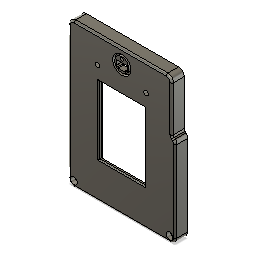
Caveatron Main Enclosure Lid v16 (Autodesk Fusion 360 design; units mm, degrees)
Autodesk Fusion 360 part; units mm, degrees
sketch "Sketch1" plane through (0, 0, 0) normal (0, 0, 1) x (1, 0, 0)
  arc A0 (6.35, 149.098) -> (3.302, 146.05) centre (6.35, 146.05) ccw
  line L0 (116.586, 156.21) -> (116.586, 152.4)
  line L1 (116.586, 152.4) -> (116.586, 105.4025)
  arc A1 (113.284, 105.4025) -> (115.1439, 100.9124) centre (119.634, 105.4025) ccw
  arc A2 (116.586, 105.4025) -> (117.4787, 103.2473) centre (119.634, 105.4025) ccw
  arc A3 (114.046, 0) -> (120.396, 6.35) centre (114.046, 6.35) ccw
  arc A4 (113.284, 146.017) -> (110.2512, 149.0649) centre (110.236, 146.017) ccw
  line L2 (97.5868, 6.35) -> (97.5868, 10.414)
  line L3 (6.35, 0) -> (23.495, 0)
  arc A5 (3.302, 16.51) -> (6.35, 13.462) centre (6.35, 16.51) ccw
  arc A6 (104.14, 156.21) -> (100.076, 160.274) centre (100.076, 156.21) ccw
  line L4 (120.396, 10.16) -> (120.396, 6.35)
  line L5 (117.4787, 103.2473) -> (118.5361, 102.1899)
  line L6 (110.236, 162.56) -> (103.886, 162.56)
  line L7 (0, 10.16) -> (0, 6.35)
  line L8 (22.8092, 6.35) -> (22.8092, 10.414)
  circle A7 centre (114.046, 6.35) radius 2.032
  arc A8 (114.3, 146.017) -> (110.2563, 150.0809) centre (110.236, 146.017) ccw
  arc A9 (114.046, 12.446) -> (118.11, 16.51) centre (114.046, 16.51) ccw
  line L9 (113.284, 146.017) -> (113.284, 105.4025)
  arc A10 (23.8252, 6.35) -> (26.8732, 3.302) centre (26.8732, 6.35) ccw
  line L10 (115.8623, 101.6308) -> (116.9197, 100.5734)
  arc A11 (116.586, 156.21) -> (110.236, 162.56) centre (110.236, 156.21) ccw
  circle A12 centre (110.236, 156.21) radius 3.81
  arc A13 (93.5228, 3.302) -> (96.5708, 6.35) centre (93.5228, 6.35) ccw
  arc A14 (22.8092, 6.35) -> (26.8732, 2.286) centre (26.8732, 6.35) ccw
  line L11 (116.586, 152.4) -> (116.586, 156.21)
  line L12 (0, 10.16) -> (0, 6.35)
  line L13 (104.14, 156.21) -> (104.14, 152.146)
  line L14 (120.396, 6.35) -> (120.396, 10.16)
  arc A15 (104.14, 152.146) -> (106.1619, 150.114) centre (106.172, 152.146) ccw
  circle A16 centre (6.35, 6.35) radius 2.032
  arc A17 (120.396, 97.6997) -> (118.5361, 102.1899) centre (114.046, 97.6997) ccw
  arc A18 (22.8092, 10.414) -> (20.7772, 12.446) centre (20.7772, 10.414) ccw
  arc A19 (0, 6.35) -> (6.35, 0) centre (6.35, 6.35) ccw
  line L15 (6.35, 0) -> (23.495, 0)
  line L16 (99.6188, 13.462) -> (114.046, 13.462)
  line L17 (20.7772, 13.462) -> (6.35, 13.462)
  arc A20 (114.3, 105.4025) -> (115.8623, 101.6308) centre (119.634, 105.4025) ccw
  arc A21 (103.124, 156.21) -> (100.076, 159.258) centre (100.076, 156.21) ccw
  line L18 (20.7772, 12.446) -> (6.35, 12.446)
  line L19 (110.2563, 150.0809) -> (106.1619, 150.114)
  line L20 (110.2512, 149.0649) -> (106.1568, 149.098)
  line L21 (96.901, 0) -> (114.046, 0)
  arc A22 (118.11, 97.6997) -> (116.9197, 100.5734) centre (114.046, 97.6997) ccw
  line L22 (103.124, 156.21) -> (103.124, 152.146)
  line L23 (23.8252, 6.35) -> (23.8252, 10.414)
  arc A23 (114.046, 13.462) -> (117.094, 16.51) centre (114.046, 16.51) ccw
  arc A24 (103.124, 152.146) -> (106.1568, 149.098) centre (106.172, 152.146) ccw
  arc A25 (99.6188, 12.446) -> (97.5868, 10.414) centre (99.6188, 10.414) ccw
  arc A26 (117.094, 97.6997) -> (116.2013, 99.855) centre (114.046, 97.6997) ccw
  arc A27 (99.6188, 13.462) -> (96.5708, 10.414) centre (99.6188, 10.414) ccw
  line L24 (115.1439, 100.9124) -> (116.2013, 99.855)
  line L25 (96.5708, 6.35) -> (96.5708, 10.414)
  line L26 (99.6188, 12.446) -> (114.046, 12.446)
  arc A28 (93.5228, 2.286) -> (97.5868, 6.35) centre (93.5228, 6.35) ccw
  line L27 (114.046, 0) -> (96.901, 0)
  arc A29 (2.286, 16.51) -> (6.35, 12.446) centre (6.35, 16.51) ccw
  line L28 (114.3, 146.017) -> (114.3, 105.4025)
  line L29 (26.8732, 3.302) -> (93.5228, 3.302)
  line L30 (23.495, 0) -> (96.901, 0)
  line L31 (26.8732, 2.286) -> (93.5228, 2.286)
  line L32 (110.236, 162.56) -> (103.886, 162.56)
  line L33 (118.11, 16.51) -> (118.11, 97.6997)
  line L34 (0, 152.4) -> (0, 10.16)
  line L35 (10.414, 150.114) -> (6.35, 150.114)
  line L36 (117.094, 16.51) -> (117.094, 97.6997)
  line L37 (10.16, 162.56) -> (6.35, 162.56)
  line L38 (3.302, 146.05) -> (3.302, 16.51)
  line L39 (100.076, 159.258) -> (16.51, 159.258)
  line L40 (2.286, 146.05) -> (2.286, 16.51)
  arc A30 (16.51, 160.274) -> (12.446, 156.21) centre (16.51, 156.21) ccw
  arc A31 (10.414, 149.098) -> (13.462, 152.146) centre (10.414, 152.146) ccw
  line L41 (10.414, 149.098) -> (6.35, 149.098)
  line L42 (0, 152.4) -> (0, 156.21)
  arc A32 (6.35, 150.114) -> (2.286, 146.05) centre (6.35, 146.05) ccw
  line L43 (13.462, 156.21) -> (13.462, 152.146)
  line L44 (0, 156.21) -> (0, 152.4)
  arc A33 (23.8252, 10.414) -> (20.7772, 13.462) centre (20.7772, 10.414) ccw
  line L45 (103.886, 162.56) -> (10.16, 162.56)
  line L46 (6.35, 162.56) -> (10.16, 162.56)
  arc A34 (16.51, 159.258) -> (13.462, 156.21) centre (16.51, 156.21) ccw
  line L47 (120.396, 10.16) -> (120.396, 97.6997)
  circle A35 centre (6.35, 156.21) radius 3.81
  line L48 (100.076, 160.274) -> (16.51, 160.274)
  arc A36 (10.414, 150.114) -> (12.446, 152.146) centre (10.414, 152.146) ccw
  arc A37 (6.35, 162.56) -> (0, 156.21) centre (6.35, 156.21) ccw
  line L49 (12.446, 156.21) -> (12.446, 152.146)
  line L50 (20.7772, 11.6332) -> (6.35, 11.6332)
  arc A38 (1.4732, 16.51) -> (6.35, 11.6332) centre (6.35, 16.51) ccw
  line L51 (1.4732, 146.05) -> (1.4732, 16.51)
  arc A39 (6.35, 150.9268) -> (1.4732, 146.05) centre (6.35, 146.05) ccw
  line L52 (10.414, 150.9268) -> (6.35, 150.9268)
  arc A40 (10.414, 150.9268) -> (11.6332, 152.146) centre (10.414, 152.146) ccw
  line L53 (11.6332, 156.21) -> (11.6332, 152.146)
  arc A41 (16.51, 161.0868) -> (11.6332, 156.21) centre (16.51, 156.21) ccw
  line L54 (100.076, 161.0868) -> (16.51, 161.0868)
  arc A42 (104.9528, 156.21) -> (100.076, 161.0868) centre (100.076, 156.21) ccw
  line L55 (104.9528, 156.21) -> (104.9528, 152.146)
  arc A43 (104.9528, 152.146) -> (106.165, 150.9268) centre (106.172, 152.146) ccw
  line L56 (110.2616, 150.8937) -> (106.165, 150.9268)
  arc A44 (115.1128, 146.017) -> (110.2616, 150.8937) centre (110.236, 146.017) ccw
  line L57 (115.1128, 146.017) -> (115.1128, 105.4025)
  arc A45 (115.1128, 105.4025) -> (116.437, 102.2056) centre (119.634, 105.4025) ccw
  line L58 (116.437, 102.2056) -> (117.4944, 101.1482)
  arc A46 (118.9228, 97.6997) -> (117.4944, 101.1482) centre (114.046, 97.6997) ccw
  line L59 (118.9228, 16.51) -> (118.9228, 97.6997)
  arc A47 (114.046, 11.6332) -> (118.9228, 16.51) centre (114.046, 16.51) ccw
  line L60 (99.6188, 11.6332) -> (114.046, 11.6332)
  arc A48 (99.6188, 11.6332) -> (98.3996, 10.414) centre (99.6188, 10.414) ccw
  line L61 (98.3996, 6.35) -> (98.3996, 10.414)
  arc A49 (93.5228, 1.4732) -> (98.3996, 6.35) centre (93.5228, 6.35) ccw
  line L62 (26.8732, 1.4732) -> (93.5228, 1.4732)
  arc A50 (21.9964, 6.35) -> (26.8732, 1.4732) centre (26.8732, 6.35) ccw
  line L63 (21.9964, 6.35) -> (21.9964, 10.414)
  arc A51 (21.9964, 10.414) -> (20.7772, 11.6332) centre (20.7772, 10.414) ccw
  line L64 (20.7772, 14.2494) -> (6.35, 14.2494)
  arc A52 (4.0894, 16.51) -> (6.35, 14.2494) centre (6.35, 16.51) ccw
  line L65 (4.0894, 146.05) -> (4.0894, 16.51)
  arc A53 (6.35, 148.3106) -> (4.0894, 146.05) centre (6.35, 146.05) ccw
  line L66 (10.414, 148.3106) -> (6.35, 148.3106)
  arc A54 (10.414, 148.3106) -> (14.2494, 152.146) centre (10.414, 152.146) ccw
  line L67 (14.2494, 156.21) -> (14.2494, 152.146)
  arc A55 (16.51, 158.4706) -> (14.2494, 156.21) centre (16.51, 156.21) ccw
  line L68 (100.076, 158.4706) -> (16.51, 158.4706)
  arc A56 (102.3366, 156.21) -> (100.076, 158.4706) centre (100.076, 156.21) ccw
  line L69 (102.3366, 156.21) -> (102.3366, 152.146)
  arc A57 (102.3366, 152.146) -> (106.1516, 148.3107) centre (106.172, 152.146) ccw
  line L70 (110.2461, 148.2776) -> (106.1516, 148.3107)
  arc A58 (112.4966, 146.017) -> (110.2461, 148.2776) centre (110.236, 146.017) ccw
  line L71 (112.4966, 146.017) -> (112.4966, 105.4025)
  arc A59 (112.4966, 105.4025) -> (114.5871, 100.3556) centre (119.634, 105.4025) ccw
  line L72 (114.5871, 100.3556) -> (115.6445, 99.2982)
  arc A60 (116.3066, 97.6997) -> (115.6445, 99.2982) centre (114.046, 97.6997) ccw
  line L73 (116.3066, 16.51) -> (116.3066, 97.6997)
  arc A61 (114.046, 14.2494) -> (116.3066, 16.51) centre (114.046, 16.51) ccw
  line L74 (99.6188, 14.2494) -> (114.046, 14.2494)
  arc A62 (99.6188, 14.2494) -> (95.7834, 10.414) centre (99.6188, 10.414) ccw
  line L75 (95.7834, 6.35) -> (95.7834, 10.414)
  arc A63 (93.5228, 4.0894) -> (95.7834, 6.35) centre (93.5228, 6.35) ccw
  line L76 (26.8732, 4.0894) -> (93.5228, 4.0894)
  arc A64 (24.6126, 6.35) -> (26.8732, 4.0894) centre (26.8732, 6.35) ccw
  line L77 (24.6126, 6.35) -> (24.6126, 10.414)
  arc A65 (24.6126, 10.414) -> (20.7772, 14.2494) centre (20.7772, 10.414) ccw
  line L78 (20.7772, 16.4338) -> (6.35, 16.4338)
  arc A66 (6.2738, 16.51) -> (6.35, 16.4338) centre (6.35, 16.51) ccw
  line L79 (6.2738, 146.05) -> (6.2738, 16.51)
  arc A67 (6.35, 146.1262) -> (6.2738, 146.05) centre (6.35, 146.05) ccw
  line L80 (10.414, 146.1262) -> (6.35, 146.1262)
  arc A68 (10.414, 146.1262) -> (16.4338, 152.146) centre (10.414, 152.146) ccw
  line L81 (16.4338, 156.21) -> (16.4338, 152.146)
  arc A69 (16.51, 156.2862) -> (16.4338, 156.21) centre (16.51, 156.21) ccw
  line L82 (100.076, 156.2862) -> (16.51, 156.2862)
  arc A70 (100.1522, 156.21) -> (100.076, 156.2862) centre (100.076, 156.21) ccw
  line L83 (100.1522, 156.21) -> (100.1522, 152.146)
  arc A71 (100.1522, 152.146) -> (106.1366, 146.1263) centre (106.172, 152.146) ccw
  line L84 (110.2351, 146.0932) -> (106.1366, 146.1263)
  arc A72 (110.3122, 146.017) -> (110.2351, 146.0932) centre (110.236, 146.017) ccw
  line L85 (110.3122, 146.017) -> (110.3122, 105.4025)
  arc A73 (110.3122, 105.4025) -> (113.0425, 98.811) centre (119.634, 105.4025) ccw
  line L86 (113.0425, 98.811) -> (114.0999, 97.7536)
  arc A74 (114.1222, 97.6997) -> (114.0999, 97.7536) centre (114.046, 97.6997) ccw
  line L87 (114.1222, 16.51) -> (114.1222, 97.6997)
  arc A75 (114.046, 16.4338) -> (114.1222, 16.51) centre (114.046, 16.51) ccw
  line L88 (99.6188, 16.4338) -> (114.046, 16.4338)
  arc A76 (99.6188, 16.4338) -> (93.599, 10.414) centre (99.6188, 10.414) ccw
  line L89 (93.599, 6.35) -> (93.599, 10.414)
  arc A77 (93.5228, 6.2738) -> (93.599, 6.35) centre (93.5228, 6.35) ccw
  line L90 (26.8732, 6.2738) -> (93.5228, 6.2738)
  arc A78 (26.797, 6.35) -> (26.8732, 6.2738) centre (26.8732, 6.35) ccw
  line L91 (26.797, 6.35) -> (26.797, 10.414)
  arc A79 (26.797, 10.414) -> (20.7772, 16.4338) centre (20.7772, 10.414) ccw
  circle A80 centre (60.198, 146.558) radius 7.9502
  circle A81 centre (60.198, 146.558) radius 10.287
  circle A82 centre (60.198, 151.892) radius 1.8796
  line L92 (53.848, 148.59) -> (66.548, 148.59)
  line L93 (66.548, 148.59) -> (66.548, 142.748)
  line L94 (66.548, 142.748) -> (53.848, 142.748)
  line L95 (53.848, 142.748) -> (53.848, 148.59)
  circle A83 centre (32.766, 132.588) radius 2.6162
  circle A84 centre (87.63, 132.588) radius 2.6162
  line L96 (6.2738, 126.238) -> (110.3122, 126.238)
  line L97 (34.29, 117.348) -> (86.106, 117.348)
  line L98 (86.106, 117.348) -> (86.106, 41.148)
  line L99 (86.106, 41.148) -> (34.29, 41.148)
  line L100 (34.29, 41.148) -> (34.29, 117.348)
  line L101 (88.646, 38.608) -> (31.75, 38.608)
  line L102 (31.75, 38.608) -> (31.75, 119.888)
  line L103 (31.75, 119.888) -> (88.646, 119.888)
  line L104 (88.646, 119.888) -> (88.646, 38.608)
  circle A85 centre (30.226, 122.428) radius 1.27
  circle A86 centre (90.17, 122.428) radius 1.27
  circle A87 centre (30.226, 27.94) radius 1.27
  circle A88 centre (90.17, 27.94) radius 1.27
  line L105 (31.75, 38.608) -> (88.646, 38.608)
  line L106 (88.646, 38.608) -> (88.646, 33.02)
  line L107 (88.646, 33.02) -> (31.75, 33.02)
  line L108 (31.75, 33.02) -> (31.75, 38.608)
  line L109 (26.416, 126.238) -> (26.416, 24.13)
  line L110 (93.98, 126.238) -> (93.98, 24.13)
  line L111 (34.29, 33.02) -> (34.29, 24.13)
  line L112 (34.29, 24.13) -> (26.416, 24.13)
  line L113 (86.106, 33.02) -> (86.106, 24.13)
  line L114 (86.106, 24.13) -> (93.98, 24.13)
  line L115 (34.29, 24.13) -> (86.106, 24.13)
  circle A89 centre (25.146, 84.328) radius 1.27
  circle A90 centre (95.25, 84.328) radius 1.27
  arc A91 (25.146, 88.138) -> (25.146, 80.518) centre (25.146, 84.328) ccw
  line L116 (25.146, 84.328) -> (25.146, 88.138) construction
  line L117 (25.146, 84.328) -> (25.146, 80.518) construction
  arc A92 (95.25, 80.518) -> (95.25, 88.138) centre (95.25, 84.328) ccw
  line L118 (95.25, 84.328) -> (95.25, 80.518) construction
  line L119 (95.25, 84.328) -> (95.25, 88.138) construction
  line L120 (95.25, 80.518) -> (93.98, 80.518)
  line L121 (95.25, 88.138) -> (93.98, 88.138)
  line L122 (25.146, 88.138) -> (26.416, 88.138)
  line L123 (25.146, 80.518) -> (26.416, 80.518)
  line L124 (34.29, 18.542) -> (86.106, 18.542)
  line L125 (86.106, 18.542) -> (86.106, 8.382)
  line L126 (86.106, 8.382) -> (34.29, 8.382)
  line L127 (34.29, 8.382) -> (34.29, 18.542)
  line L128 (26.416, 24.13) -> (26.416, 12.5216)
  line L129 (34.29, 24.13) -> (34.29, 18.542)
  line L130 (86.106, 24.13) -> (86.106, 18.542)
  line L131 (93.98, 24.13) -> (93.98, 12.5216)
  line L132 (34.29, 32.004) -> (86.106, 32.004)
  line L133 (81.28, 138.938) -> (93.98, 138.938)
  line L134 (93.98, 138.938) -> (93.98, 126.238)
  line L135 (93.98, 126.238) -> (81.28, 126.238)
  line L136 (81.28, 126.238) -> (81.28, 138.938)
  line L137 (81.28, 138.938) -> (93.98, 126.238) construction
  line L138 (93.98, 138.938) -> (81.28, 126.238) construction
  line L139 (26.416, 138.938) -> (39.116, 138.938)
  line L140 (39.116, 138.938) -> (39.116, 126.238)
  line L141 (39.116, 126.238) -> (26.416, 126.238)
  line L142 (26.416, 126.238) -> (26.416, 138.938)
  line L143 (26.416, 138.938) -> (39.116, 126.238) construction
  line L144 (39.116, 138.938) -> (26.416, 126.238) construction
  circle A93 centre (114.046, 6.35) radius 3.81
  circle A94 centre (6.35, 6.35) radius 3.81
  line L145 (64.262, 142.748) -> (56.134, 142.748)
  line L146 (56.134, 142.748) -> (56.134, 141.224)
  line L147 (56.134, 141.224) -> (64.262, 141.224)
  line L148 (64.262, 141.224) -> (64.262, 142.748)
  point P0 (87.63, 132.588)
  point P1 (32.766, 132.588)
  dimension "d2" = 10.16
  dimension "d3" = 23.495
  dimension "d5" = 6.35
  dimension "d6" = 3.048
  dimension "d7" = 6.35
  dimension "d8" = 6.35
  dimension "d9" = 6.35
  dimension "d10" = 6.35
  dimension "d11" = 3.048
  dimension "d12" = 3.048
  dimension "d13" = 3.048
  dimension "d14" = 3.048
  dimension "d15" = 3.048
  dimension "d16" = 3.048
  dimension "d17" = 3.048
  dimension "d18" = 3.048
  dimension "d19" = 3.048
  dimension "d20" = 3.048
  dimension "d21" = 3.048
  dimension "d22" = 3.048
  dimension "d30" = 7.62
  dimension "d31" = 7.62
  dimension "d32" = 4.064
  dimension "d33" = 4.064
  dimension "d40" = 0.8128
  dimension "d41" = -0.7874
  dimension "d42" = -2.9718
  dimension "d43" = 15.9004
  dimension "d44" = 60.198
  dimension "d45" = 16.002
  dimension "d46" = 2.3368
  dimension "d47" = 3.7592
  dimension "d48" = 5.334
  dimension "d49" = 12.7
  dimension "d50" = 5.842
  dimension "d51" = 6.35
  dimension "d52" = 3.302
  dimension "d53" = 5.2324
  dimension "d54" = 32.766
  dimension "d55" = 5.2324
  dimension "d56" = 54.864
  dimension "d57" = 29.972
  dimension "d58" = 29.972
  dimension "d59" = 36.322
  dimension "d60" = 51.816
  dimension "d61" = 76.2
  dimension "d62" = 34.29
  dimension "d63" = 41.148
  dimension "d64" = -2.54
  dimension "d65" = 2.54
  dimension "d66" = 4.064
  dimension "d67" = 5.08
  dimension "d68" = 2.54
  dimension "d69" = 4.064
  dimension "d70" = 5.08
  dimension "d71" = 2.54
  dimension "d72" = 4.064
  dimension "d73" = 13.208
  dimension "d74" = 2.54
  dimension "d75" = 13.208
  dimension "d76" = 4.064
  dimension "d77" = 5.588
  dimension "d78" = 102.108
  dimension "d79" = 7.874
  dimension "d80" = 102.108
  dimension "d81" = 7.874
  dimension "d82" = 2.54
  dimension "d83" = 33.02
  dimension "d84" = 9.144
  dimension "d85" = 2.54
  dimension "d86" = 33.02
  dimension "d87" = 9.144
  dimension "d88" = 3.81
  dimension "d89" = 180
  dimension "d90" = 3.81
  dimension "d91" = 180
  dimension "d92" = 10.16
  dimension "d93" = 5.08
  dimension "d108" = 4.064
  dimension "d121" = 12.7
  dimension "d122" = 12.7
  dimension "d123" = 12.7
  dimension "d124" = 12.7
  dimension "d132" = 7.62
  dimension "d133" = 7.62
  dimension "d170" = 8.128
  dimension "d171" = 1.524
  dimension "d172" = 2.286
  dimension "d175" = 26.797
  dimension "d176" = 26.797
  constraint horizontal L15
  constraint vertical L14
  constraint horizontal L6
  constraint vertical L44
  constraint vertical L0
  constraint horizontal L46
  constraint vertical L42
  constraint horizontal L32
  constraint vertical L11
  constraint horizontal L3
  constraint vertical L12
  constraint horizontal L27
  constraint vertical L4
  constraint tangent L5 A17
  constraint tangent A17 L47
  constraint tangent A2 L5
  constraint tangent L1 A2
  constraint tangent L6 A11
  constraint tangent L0 A11
  constraint tangent L46 A37
  constraint tangent L44 A37
  constraint tangent A3 L27
  constraint tangent A3 L4
  constraint tangent L3 A19
  constraint tangent L7 A19
  constraint parallel L34 L38
  constraint parallel L29 L30
  constraint parallel L36 L47
  constraint concentric A17 A26
  constraint parallel L5 L24
  constraint concentric A1 A2
  constraint parallel L1 L9
  constraint parallel L39 L45
  constraint tangent A26 L24
  constraint tangent A1 L9
  constraint tangent A1 L24
  constraint tangent A26 L36
  constraint tangent A0 L38
  constraint tangent A0 L41
  constraint tangent A31 L41
  constraint tangent A31 L43
  constraint tangent L43 A34
  constraint tangent L39 A34
  constraint tangent A21 L39
  constraint tangent A21 L22
  constraint tangent L22 A24
  constraint tangent A4 L9
  constraint tangent L16 A23
  constraint tangent A23 L36
  constraint tangent L16 A27
  constraint tangent A27 L25
  constraint tangent A13 L29
  constraint tangent A13 L25
  constraint tangent A10 L29
  constraint tangent A10 L23
  constraint tangent L17 A33
  constraint tangent L23 A33
  constraint tangent A5 L17
  constraint tangent A5 L38
  constraint parallel L17 L18
  constraint concentric A5 A29
  constraint parallel L38 L40
  constraint concentric A0 A32
  constraint parallel L35 L41
  constraint concentric A31 A36
  constraint parallel L43 L49
  constraint concentric A30 A34
  constraint parallel L39 L48
  constraint concentric A6 A21
  constraint parallel L13 L22
  constraint concentric A15 A24
  constraint concentric A4 A8
  constraint parallel L9 L28
  constraint concentric A1 A20
  constraint parallel L10 L24
  constraint concentric A22 A26
  constraint parallel L33 L36
  constraint concentric A9 A23
  constraint parallel L16 L26
  constraint concentric A25 A27
  constraint parallel L2 L25
  constraint concentric A13 A28
  constraint parallel L29 L31
  constraint concentric A10 A14
  constraint parallel L8 L23
  constraint concentric A18 A33
  constraint tangent L8 A18
  constraint tangent L8 A14
  constraint tangent A28 L31
  constraint tangent L2 A28
  constraint tangent A9 L26
  constraint tangent A9 L33
  constraint tangent L10 A22
  constraint tangent A25 L26
  constraint tangent L10 A20
  constraint tangent A29 L40
  constraint tangent A6 L13
  constraint tangent A30 L48
  constraint tangent L13 A15
  constraint tangent A36 L49
  constraint tangent A6 L48
  constraint tangent A22 L33
  constraint tangent L2 A25
  constraint tangent A14 L31
  constraint tangent L35 A36
  constraint tangent L35 A32
  constraint tangent L40 A32
  constraint tangent L18 A29
  constraint tangent A8 L28
  constraint tangent A30 L49
  constraint tangent A20 L28
  constraint tangent A18 L18
  constraint concentric A35 A37
  constraint concentric A11 A12
  constraint concentric A3 A7
  constraint concentric A16 A19
  constraint horizontal L92
  constraint vertical L93
  constraint horizontal L94
  constraint vertical L95
  constraint coincident L79 L96.start
  constraint coincident L85 L96.end
  constraint perpendicular L85 L96
  constraint horizontal L97
  constraint vertical L98
  constraint horizontal L99
  constraint vertical L100
  constraint horizontal L105
  constraint vertical L106
  constraint horizontal L107
  constraint vertical L108
  constraint coincident L96 L109.start
  constraint perpendicular L96 L109
  constraint coincident L96 L110.start
  constraint perpendicular L96 L110
  constraint coincident L107 L111.start
  constraint perpendicular L107 L111
  constraint perpendicular L109 L112
  constraint coincident L107 L113.start
  constraint perpendicular L107 L113
  constraint perpendicular L110 L114
  constraint coincident A89.centre A91.centre
  constraint coincident A90.centre A92.centre
  constraint coincident L110 L120.end
  constraint tangent A92 L120
  constraint perpendicular L110 L120
  constraint coincident L110 L121.end
  constraint tangent A92 L121
  constraint coincident L109 L122.end
  constraint tangent A91 L122
  constraint perpendicular L109 L122
  constraint coincident L109 L123.end
  constraint tangent A91 L123
  constraint horizontal L124
  constraint vertical L125
  constraint horizontal L126
  constraint vertical L127
  constraint coincident A79 L128.end
  constraint perpendicular L112 L128
  constraint perpendicular L124 L129
  constraint perpendicular L124 L130
  constraint coincident A76 L131.end
  constraint perpendicular L114 L131
  constraint coincident L111 L132.start
  constraint coincident L113 L132.end
  constraint perpendicular L113 L132
  constraint perpendicular L133 L134
  constraint parallel L133 L135
  constraint parallel L134 L136
  constraint horizontal L133
  constraint coincident L137 L3 P0
  constraint coincident L138 P0
  constraint coincident P0 A84.centre
  constraint perpendicular L139 L140
  constraint parallel L139 L141
  constraint parallel L140 L142
  constraint horizontal L139
  constraint coincident L143 P1
  constraint coincident L144 P1
  constraint coincident P1 A83.centre
  constraint concentric A7 A93
  constraint concentric A19 A94
  constraint horizontal L145
  constraint vertical L146
  constraint horizontal L147
  constraint vertical L148
  constraint coincident L94 L145.start
  measures "d2" distance of L7.start origin
  measures "d3" distance of L3.end origin
  measures "d5" radius of A17
  measures "d6" radius of A2
  measures "d7" radius of A11
  measures "d8" radius of A37
  measures "d9" radius of A3
  measures "d10" radius of A19
  measures "d11" radius of A0
  measures "d12" radius of A31
  measures "d13" radius of A34
  measures "d14" radius of A21
  measures "d15" radius of A24
  measures "d16" radius of A4
  measures "d17" radius of A23
  measures "d18" radius of A27
  measures "d19" radius of A13
  measures "d20" radius of A10
  measures "d21" radius of A33
  measures "d22" radius of A5
  measures "d30" diameter of A35
  measures "d31" diameter of A12
  measures "d32" diameter of A7
  measures "d33" diameter of A16
  measures "d43" diameter of A80
  measures "d44" distance of L34 A80.centre
  measures "d45" distance of L45 A80.centre
  measures "d47" diameter of A82
  measures "d48" distance of A80.centre A82.centre
  measures "d49" distance of L92.start L92.end
  measures "d50" distance of L92.start L94.end
  measures "d51" distance of A80.centre L93
  measures "d52" distance of A82.centre L92
  measures "d53" diameter of A83
  measures "d54" distance of L34 P1
  measures "d55" diameter of A84
  measures "d56" horizontal distance of P1 P0
  measures "d57" distance of L45 P1
  measures "d58" distance of L45 P0
  measures "d59" distance of L45 L96
  measures "d60" distance of L97.start L97.end
  measures "d61" distance of L97.start L99.end
  measures "d62" distance of L34 L100
  measures "d63" distance of L30 L99
  measures "d65" diameter of A85
  measures "d66" distance of L100 A85.centre
  measures "d67" distance of L97 A85.centre
  measures "d68" diameter of A86
  measures "d69" distance of L98 A86.centre
  measures "d70" distance of L97 A86.centre
  measures "d71" diameter of A87
  measures "d72" distance of L100 A87.centre
  measures "d73" distance of L99 A87.centre
  measures "d74" diameter of A88
  measures "d75" distance of L99 A88.centre
  measures "d76" distance of L98 A88.centre
  measures "d77" distance of L101.end L107.end
  measures "d78" distance of L109.start L109.end
  measures "d79" distance of L100 L109
  measures "d80" distance of L110.start L110.end
  measures "d81" distance of L98 L110
  measures "d82" diameter of A89
  measures "d83" distance of L97 A89.centre
  measures "d84" distance of L100 A89.centre
  measures "d85" diameter of A90
  measures "d86" distance of L97 A90.centre
  measures "d87" distance of L98 A90.centre
  measures "d88" radius of A91
  measures "d89" angle of L116 L117
  measures "d90" radius of A92
  measures "d91" angle of L118 L119
  measures "d92" distance of L124.start L126.end
  measures "d93" distance of L17 L124
  measures "d108" distance of A87.centre L132
  measures "d121" distance of L110.start L135.end
  measures "d122" distance of L133.end L110.start
  measures "d123" distance of L140.end L109.start
  measures "d124" distance of L139.end L140.end
  measures "d132" diameter of A93
  measures "d133" diameter of A94
  measures "d170" distance of L145.start L145.end
  measures "d171" distance of L145.start L147.end
  measures "d172" distance of L93 L148
  measures "d175" distance of L4 L89
  measures "d176" distance of L7 L91
extrude "Extrude1" add sketch "Sketch1" against normal blind 13.97 contours L0 L1 A2 A3 L3 L4 L5 L6 L7 A11 L11 L12 L14 A17 A19 L15 L21 L27 L30 L32 L34 L37 L42 L44 L45 L46 L47 A37 | L64 A52 L65 A53 L66 A54 L67 A55 L68 A56 L69 A57 L70 A58 L71 A59 L72 A60 L73 A61 L74 A62 L75 A63 L76 A64 L77 A65 | A93 | A94 makes body 1 at (0, 56.3033, -4.6567) makes body 2 at (6.2738, 102.87, -4.6567)
extrude "Extrude2" add sketch "Sketch1" against normal blind 10.922 contours A0 A1 A4 A5 L9 A10 A13 L16 L17 A21 L20 L22 L23 A23 A24 A26 A27 L24 L25 L29 L36 L38 L39 A31 L41 L43 A33 A34 | L2 A6 L8 A8 A9 L10 A14 L13 A15 A18 A20 L18 L19 A22 A25 L26 A28 A29 L28 L31 L33 L35 L40 A30 A32 L48 A36 L49 | L50 A38 L51 A39 L52 A40 L53 A41 L54 A42 L55 A43 L56 A44 L57 A45 L58 A46 L59 A47 L60 A48 L61 A49 L62 A50 L63 A51 bodies 1 2
extrude "Extrude3" add sketch "Sketch1" against normal blind 3.048 contours L78 A66 L79 A79 L96 L109 A91 L122 L123 L128 | L85 A73 L86 A74 L87 A75 L88 A76 L96 L110 A92 L120 L121 L131 bodies 1
extrude "Extrude4" add sketch "Sketch1" against normal blind 4.572 separate body contours L124 L125 L126 L127 makes body 3
extrude "Extrude5" add sketch "Sketch1" against normal blind 13.97 contours L82 A81 picked at (60.4249, 156.465) bodies 1
extrude "Extrude6" add sketch "Sketch1" against normal blind 6.096 contours L79 A67 L80 A68 L81 A69 L82 A70 L83 A71 L84 A72 L85 A81 L96 L133 L134 L136 L139 L140 L142 | L96 L139 L140 L141 L142 | L96 L133 L134 L135 L136 | L82 A81 | A80 | L94 L145 L146 L147 L148 | A83 | A84 picked at (60, 155.6861) bodies 1
extrude "Extrude7" cut sketch "Sketch1" against normal blind 3.048 contours L82 A81 | L82 A81 bodies 1
extrude "Extrude8" add sketch "Sketch1" against normal blind 7.112 contours L96 L102 L103 L104 L106 L107 L108 L109 L110 L111 L112 L113 L114 L135 L141 | L109 A91 L122 L123 | L110 A92 L120 L121 bodies 1
extrude "Extrude9" add sketch "Sketch1" against normal blind 3.048 contours L107 L111 L113 L132 | L101 L105 L106 L107 L108 | L101 L102 L103 L104 L105 bodies 1
extrude "Extrude10" add sketch "Sketch1" against normal blind 3.048 contours L111 L113 L115 L132 bodies 1
extrude "Extrude11" add sketch "Sketch1" against normal blind 4.572 contours A76 L89 A77 L90 A78 L91 A79 L112 L114 L125 L126 L127 L128 L129 L130 L131 | L115 L124 L129 L130 bodies 1 3
extrude "Extrude12" add sketch "Sketch1" against normal blind 2.032 contours A85 | A86 | A87 | A88 bodies 1
extrude "Extrude13" add sketch "Sketch1" against normal blind 3.048 contours A89 | A90 bodies 1
extrude "Extrude14" add sketch "Sketch1" against normal blind 10.16 contours L96 L139 L140 L141 L142 | L96 L133 L134 L135 L136 | A83 | A84 bodies 1
sketch "Sketch2" plane through (0, 0, -6.096) normal (0, 0, -1) x (-1, 0, 0)
  line L0 (-81.28, 138.938) -> (-81.28, 126.238)
  line L1 (-81.28, 126.238) -> (-39.116, 126.238)
  line L2 (-39.116, 126.238) -> (-39.116, 138.938)
  line L3 (-39.116, 138.938) -> (-26.416, 138.938)
  line L4 (-26.416, 138.938) -> (-26.416, 126.238)
  line L5 (-26.416, 126.238) -> (-6.2738, 126.238)
  line L6 (-6.2738, 126.238) -> (-6.2738, 146.05)
  arc A0 (-6.2738, 146.05) -> (-6.35, 146.1262) centre (-6.35, 146.05) ccw
  line L7 (-6.35, 146.1262) -> (-10.414, 146.1262)
  arc A1 (-16.4338, 152.146) -> (-10.414, 146.1262) centre (-10.414, 152.146) ccw
  line L8 (-16.4338, 152.146) -> (-16.4338, 156.21)
  arc A2 (-16.4338, 156.21) -> (-16.51, 156.2862) centre (-16.51, 156.21) ccw
  line L9 (-16.51, 156.2862) -> (-100.076, 156.2862)
  arc A3 (-100.076, 156.2862) -> (-100.1522, 156.21) centre (-100.076, 156.21) ccw
  line L10 (-100.1522, 156.21) -> (-100.1522, 152.146)
  arc A4 (-106.1366, 146.1263) -> (-100.1522, 152.146) centre (-106.172, 152.146) ccw
  line L11 (-106.1366, 146.1263) -> (-110.2351, 146.0932)
  arc A5 (-110.2351, 146.0932) -> (-110.3122, 146.017) centre (-110.236, 146.017) ccw
  line L12 (-110.3122, 146.017) -> (-110.3122, 126.238)
  line L13 (-93.98, 126.238) -> (-93.98, 138.938)
  line L14 (-93.98, 138.938) -> (-81.28, 138.938)
  line L15 (-53.848, 142.748) -> (-66.548, 142.748)
  line L16 (-66.548, 142.748) -> (-66.548, 148.59)
  line L17 (-66.548, 148.59) -> (-53.848, 148.59)
  line L18 (-53.848, 148.59) -> (-53.848, 142.748)
  circle A6 centre (-60.198, 151.892) radius 1.8796
  line L19 (-57.9103, 147.9296) -> (-55.6226, 151.892)
  line L20 (-55.6226, 151.892) -> (-57.9103, 155.8544)
  line L21 (-57.9103, 155.8544) -> (-62.4857, 155.8544)
  line L22 (-62.4857, 155.8544) -> (-64.7734, 151.892)
  line L23 (-64.7734, 151.892) -> (-62.4857, 147.9296)
  line L24 (-62.4857, 147.9296) -> (-57.9103, 147.9296)
  line L25 (-66.548, 148.59) -> (-53.848, 148.59)
  line L26 (-53.848, 148.59) -> (-53.848, 156.2862)
  line L27 (-53.848, 156.2862) -> (-66.548, 156.2862)
  line L28 (-66.548, 156.2862) -> (-66.548, 148.59)
  line L29 (-110.3122, 126.238) -> (-93.98, 126.238)
  point P0 (-60.198, 151.892)
  dimension "d127" = 3.9624
  constraint coincident P0 A6.centre
  constraint horizontal L25
  constraint vertical L26
  constraint horizontal L27
  constraint vertical L28
  constraint coincident L9 L26.end
  constraint coincident L16.end L17.start
  measures "d127" distance of P0 L24
extrude "Extrude15" add sketch "Sketch2" along normal blind 3.048 contours L9 L17 L19 L20 L21 L22 L23 L25 L26 L27 L28 bodies 1
sketch "Sketch3" plane through (0, 0, -13.97) normal (0, 0, -1) x (-1, 0, 0)
  circle A0 centre (-6.35, 6.35) radius 2.032
  arc A1 (-26.8732, 1.4732) -> (-21.9964, 6.35) centre (-26.8732, 6.35) ccw
  line L0 (-26.8732, 1.4732) -> (-93.5228, 1.4732)
  arc A2 (-98.3996, 6.35) -> (-93.5228, 1.4732) centre (-93.5228, 6.35) ccw
  line L1 (-98.3996, 6.35) -> (-98.3996, 10.414)
  arc A3 (-98.3996, 10.414) -> (-99.6188, 11.6332) centre (-99.6188, 10.414) ccw
  line L2 (-99.6188, 11.6332) -> (-114.046, 11.6332)
  arc A4 (-118.9228, 16.51) -> (-114.046, 11.6332) centre (-114.046, 16.51) ccw
  line L3 (-118.9228, 16.51) -> (-118.9228, 97.6997)
  arc A5 (-117.4944, 101.1482) -> (-118.9228, 97.6997) centre (-114.046, 97.6997) ccw
  line L4 (-117.4944, 101.1482) -> (-116.437, 102.2056)
  arc A6 (-116.437, 102.2056) -> (-115.1128, 105.4025) centre (-119.634, 105.4025) ccw
  line L5 (-115.1128, 105.4025) -> (-115.1128, 146.017)
  arc A7 (-110.2616, 150.8937) -> (-115.1128, 146.017) centre (-110.236, 146.017) ccw
  line L6 (-110.2616, 150.8937) -> (-106.165, 150.9268)
  arc A8 (-106.165, 150.9268) -> (-104.9528, 152.146) centre (-106.172, 152.146) ccw
  line L7 (-104.9528, 152.146) -> (-104.9528, 156.21)
  arc A9 (-100.076, 161.0868) -> (-104.9528, 156.21) centre (-100.076, 156.21) ccw
  line L8 (-100.076, 161.0868) -> (-16.51, 161.0868)
  arc A10 (-11.6332, 156.21) -> (-16.51, 161.0868) centre (-16.51, 156.21) ccw
  line L9 (-11.6332, 156.21) -> (-11.6332, 152.146)
  arc A11 (-11.6332, 152.146) -> (-10.414, 150.9268) centre (-10.414, 152.146) ccw
  line L10 (-10.414, 150.9268) -> (-6.35, 150.9268)
  arc A12 (-1.4732, 146.05) -> (-6.35, 150.9268) centre (-6.35, 146.05) ccw
  line L11 (-1.4732, 146.05) -> (-1.4732, 16.51)
  arc A13 (-6.35, 11.6332) -> (-1.4732, 16.51) centre (-6.35, 16.51) ccw
  line L12 (-6.35, 11.6332) -> (-20.7772, 11.6332)
  arc A14 (-20.7772, 11.6332) -> (-21.9964, 10.414) centre (-20.7772, 10.414) ccw
  line L13 (-21.9964, 10.414) -> (-21.9964, 6.35)
  circle A15 centre (-6.35, 156.21) radius 3.81
  circle A16 centre (-110.236, 156.21) radius 3.81
  circle A17 centre (-114.046, 6.35) radius 2.032
  line L14 (-116.586, 156.21) -> (-116.586, 105.4025)
  arc A18 (-117.4787, 103.2473) -> (-116.586, 105.4025) centre (-119.634, 105.4025) ccw
  line L15 (-117.4787, 103.2473) -> (-118.5361, 102.1899)
  arc A19 (-118.5361, 102.1899) -> (-120.396, 97.6997) centre (-114.046, 97.6997) ccw
  line L16 (-120.396, 97.6997) -> (-120.396, 6.35)
  arc A20 (-120.396, 6.35) -> (-114.046, 0) centre (-114.046, 6.35) ccw
  line L17 (-114.046, 0) -> (-6.35, 0)
  arc A21 (-6.35, 0) -> (0, 6.35) centre (-6.35, 6.35) ccw
  line L18 (0, 6.35) -> (0, 156.21)
  arc A22 (0, 156.21) -> (-6.35, 162.56) centre (-6.35, 156.21) ccw
  line L19 (-6.35, 162.56) -> (-110.236, 162.56)
  arc A23 (-110.236, 162.56) -> (-116.586, 156.21) centre (-110.236, 156.21) ccw
  circle A24 centre (-6.35, 156.21) radius 2.6162
  circle A25 centre (-110.236, 156.21) radius 2.6162
  line L20 (-19.812, 7.874) -> (-11.684, 7.874)
  line L21 (-11.684, 7.874) -> (-11.684, 4.572)
  line L22 (-11.684, 4.572) -> (-19.812, 4.572)
  line L23 (-19.812, 4.572) -> (-19.812, 7.874)
  line L24 (-108.712, 7.874) -> (-100.584, 7.874)
  line L25 (-100.584, 7.874) -> (-100.584, 4.572)
  line L26 (-100.584, 4.572) -> (-108.712, 4.572)
  line L27 (-108.712, 4.572) -> (-108.712, 7.874)
  dimension "d130" = 5.2324
  dimension "d131" = 5.2324
  dimension "d152" = 8.128
  dimension "d153" = 3.302
  dimension "d154" = 11.684
  dimension "d155" = 4.572
  dimension "d156" = 8.128
  dimension "d157" = 3.302
  dimension "d158" = 11.684
  dimension "d159" = 4.572
  constraint concentric A15 A24
  constraint concentric A16 A25
  constraint horizontal L20
  constraint vertical L21
  constraint horizontal L22
  constraint vertical L23
  constraint horizontal L24
  constraint vertical L25
  constraint horizontal L26
  constraint vertical L27
  measures "d130" diameter of A24
  measures "d131" diameter of A25
  measures "d152" distance of L20.start L20.end
  measures "d153" distance of L20.start L22.end
  measures "d154" distance of L18 L21
  measures "d155" distance of L17 L22
  measures "d156" distance of L24.start L24.end
  measures "d157" distance of L24.start L26.end
  measures "d158" distance of L16 L27
  measures "d159" distance of L17 L26
extrude "Extrude16" cut sketch "Sketch1" against normal blind 4.572 contours A93 | A94 bodies 1
chamfer "Chamfer1" distance 2.0574 distance2 1.778 1 edges at (4.4555, 5.6152, -4.572) measured on face at (8.3719, 6.1477, -7.7047) on bodies 1
chamfer "Chamfer2" distance 2.0574 distance2 1.778 1 edges at (112.1515, 5.6152, -4.572) measured on face at (114.0967, 8.3814, -10.8373) on bodies 1
extrude "Extrude17" add sketch "Sketch1" against normal blind 13.97 contours A12 | A35 bodies 1
extrude "Extrude18" cut sketch "Sketch3" against normal blind 6.604 contours A24 | A25 bodies 1
extrude "Extrude19" cut sketch "Sketch1" against normal blind 6.604 contours A83 | A84 bodies 1
draft "Draft1" angle 2.41 neutral plane through (0, 0, -13.97) pull (0, 0, -1) 2 faces at (3.7371, 156.0796, -9.5673) (107.6231, 156.0796, -9.5673) on bodies 1
draft "Draft2" angle 2.41 neutral plane through (0, 0, 0) pull (0, 0, 1) 2 faces at (35.3789, 132.4576, -4.4027) (85.0268, 132.3275, -4.4027) on bodies 1
fillet "Fillet1" radius 2.032 12 edges at (58.293, 162.56, 0) (1.8599, 160.7001, 0) (0, 81.28, 0) (1.8599, 1.8599, 0) (60.198, 0, 0) (118.5361, 1.8599, 0) (120.396, 52.0249, 0) (119.9126, 100.1298, 0) (118.0074, 102.7186, 0) (116.818, 104.2361, 0) (116.586, 130.8063, 0) (114.7261, 160.7001, 0) on bodies 1
fillet "Fillet2" radius 1.27 4 edges at (60.198, 117.348, 0) (86.106, 79.248, 0) (60.198, 41.148, 0) (34.29, 79.248, 0) on bodies 1
extrude "Extrude20" cut sketch "Sketch3" against normal blind 9.652 contours L20 L21 L22 L23 | L24 L25 L26 L27 bodies 1
sketch "Sketch4" plane through (0, 0, 0) normal (0, -1, 0) x (1, 0, 0)
  line L0 (114.046, -2.032) -> (6.35, -2.032)
  line L1 (6.35, -2.032) -> (6.35, -13.97)
  line L2 (6.35, -13.97) -> (114.046, -13.97)
  line L3 (114.046, -13.97) -> (114.046, -2.032)
  circle A0 centre (104.648, -9.144) radius 2.032
  line L4 (120.396, -2.032) -> (120.396, -13.97)
  line L5 (114.046, -13.97) -> (6.35, -13.97)
  circle A1 centre (15.748, -9.144) radius 2.032
  line L6 (0, -2.032) -> (0, -13.97)
  dimension "d162" = 4.064
  dimension "d163" = 15.748
  dimension "d164" = 4.826
  dimension "d165" = 4.064
  dimension "d166" = 4.826
  dimension "d167" = 15.748
  measures "d162" diameter of A0
  measures "d163" distance of A0.centre L4
  measures "d164" distance of A0.centre L5
  measures "d165" diameter of A1
  measures "d166" distance of L5 A1.centre
  measures "d167" distance of A1.centre L6
extrude "Extrude21" cut sketch "Sketch4" against normal blind 9.398 contours A0 | A1 bodies 1
extrude "Extrude22" cut sketch "Sketch1" against normal blind 6.35 contours L94 L145 L146 L147 L148 bodies 1
extrude "Extrude23" add sketch "Sketch1" against normal blind 6.477 contours L124 L125 L126 L127 bodies 1
